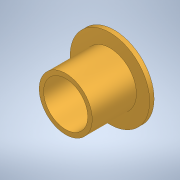
# Autodesk Inventor part: オイレスドライメットFd10D12L11
Saved by Autodesk Inventor 2020.2 (Build 242310000, 310)
## iProperties
Created: 2020-04-13
Part Number: オイレスドライメットFd10D12L11
Material: アセタール樹脂、黒
Document SubType Name: Modeling
Designer: aoyama
Density: 1.425 g/cm^3
Appearance: 真鍮 - サテン
Author: aoyama
Autodesk Inventor part; units mm, degrees
ref_plane "YZ Plane" through (0, 0, 0) normal (1, 0, 0) x (0, 1, 0)
ref_plane "XZ Plane" through (0, 0, 0) normal (0, 1, 0) x (-1, 0, 0)
ref_plane "XY Plane" through (0, 0, 0) normal (0, 0, 1) x (1, 0, 0)
sketch "スケッチ1" plane through (0, 0, 0) normal (0, 0, 1) x (1, 0, 0)
  circle A0 centre (0, 0) radius 5
  circle A1 centre (0, 0) radius 6
  circle A2 centre (0, 0) radius 9
  dimension "d0" = 10
  dimension "d1" = 12
  dimension "d2" = 18
  constraints: 3 centre point, 3 coincident
  measures "d0" diameter of A0
  measures "d1" diameter of A1
  measures "d2" diameter of A2
extrude "押し出し1" add sketch "スケッチ1" along normal blind 1 contours A2
extrude "押し出し2" add sketch "スケッチ1" along normal blind 11 contours A1
